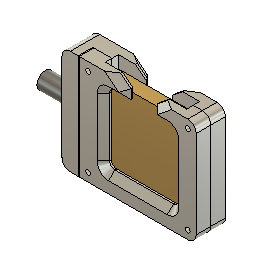
Elara 4th axis 0.5in jig (Autodesk Fusion 360 design; units mm, degrees)
Autodesk Fusion 360 part; units mm, degrees
note: some values were not read from the file. Set by a fixed rule: which sketch regions a step uses.
sketch "Sketch1" plane through (0, 0, 0) normal (0, 0, 1) x (1, 0, 0)
  line L0 (8, 0) -> (120.4, 0)
  line L1 (128.4, 8) -> (128.4, 92)
  line L2 (120.4, 100) -> (8, 100)
  line L3 (0, 92) -> (0, 8)
  circle A0 centre (72.7, 50) radius 23.3625 construction
  circle A1 centre (72.7, 50) radius 18.6 construction
  circle A2 centre (72.7, 50) radius 24
  line L4 (44.6, 83.1) -> (100.8, 83.1)
  line L5 (105.8, 78.1) -> (105.8, 21.9)
  line L6 (100.8, 16.9) -> (44.6, 16.9)
  line L7 (39.6, 21.9) -> (39.6, 78.1)
  arc A3 (128.4, 92) -> (120.4, 100) centre (120.4, 92) ccw
  arc A4 (120.4, 0) -> (128.4, 8) centre (120.4, 8) ccw
  circle A5 centre (120.4, 92) radius 1.65
  circle A6 centre (120.4, 8) radius 1.65
  circle A7 centre (25, 92) radius 1.65
  circle A8 centre (25, 8) radius 1.65
  line L8 (0, 50) -> (-50, 50) construction
  line L9 (60.2, 70.4878) -> (60.2, 100)
  line L10 (85.2, 70.4878) -> (85.2, 100)
  line L11 (72.7, 50) -> (72.7, 100) construction
  line L12 (16, 100) -> (16, 0)
  line L13 (0, 58) -> (-30, 58)
  line L14 (-30, 58) -> (-30, 50)
  line L15 (-30, 50) -> (0, 50)
  line L16 (33.8, 0) -> (33.8, 100)
  line L17 (111.6, 0) -> (111.6, 100)
  line L18 (15.5, 0) -> (15.5, 100)
  line L19 (16.5, 0) -> (16.5, 100)
  circle A9 centre (25, 92) radius 2.25
  circle A10 centre (120.4, 92) radius 2.25
  circle A11 centre (120.4, 8) radius 2.25
  circle A12 centre (25, 8) radius 2.25
  line L20 (60.2, 92) -> (50.2, 100)
  line L21 (85.2, 92) -> (95.2, 100)
  line L22 (34.6, 100) -> (34.6, 0)
  line L23 (110.8, 0) -> (110.8, 100)
  line L24 (33.8, 11.9) -> (111.6, 11.9)
  line L25 (33.8, 88.1) -> (111.6, 88.1)
  arc A13 (33.8, 11.9) -> (43.8, 11.9) centre (38.8, 11.9) ccw
  arc A14 (101.6, 11.9) -> (111.6, 11.9) centre (106.6, 11.9) ccw
  arc A15 (8, 100) -> (0, 92) centre (8, 92) ccw
  arc A16 (0, 8) -> (8, 0) centre (8, 8) ccw
  line L26 (103.9728, 65.6083) -> (118.9039, 65.6806) construction
  line L27 (118.9039, 65.6806) -> (118.8893, 68.6863) construction
  line L28 (118.8893, 68.6863) -> (103.9583, 68.614) construction
  line L29 (103.9583, 68.614) -> (103.9728, 65.6083) construction
  line L30 (0.7334, -6.4335) -> (20.3258, -6.3506) construction
  line L31 (20.3258, -6.3506) -> (20.3131, -3.3448) construction
  line L32 (20.3131, -3.3448) -> (0.7207, -3.4278) construction
  line L33 (0.7207, -3.4278) -> (0.7334, -6.4335) construction
  line L34 (-18.6738, 11.9015) -> (0.9186, 11.9844) construction
  line L35 (0.9186, 11.9844) -> (0.9059, 14.9901) construction
  line L36 (0.9059, 14.9901) -> (-18.6865, 14.9072) construction
  line L37 (-18.6865, 14.9072) -> (-18.6738, 11.9015) construction
  line L38 (-9.6516, 2.3848) -> (13.035, 2.4962) construction
  line L39 (13.035, 2.4962) -> (13.0067, 8.2636) construction
  line L40 (13.0067, 8.2636) -> (-9.6799, 8.1522) construction
  line L41 (-9.6799, 8.1522) -> (-9.6516, 2.3848) construction
  line L42 (0, 50) -> (22, 50) construction
  arc A17 (44.6, 83.1) -> (39.6, 78.1) centre (44.6, 78.1) ccw
  arc A18 (105.8, 78.1) -> (100.8, 83.1) centre (100.8, 78.1) ccw
  arc A19 (100.8, 16.9) -> (105.8, 21.9) centre (100.8, 21.9) ccw
  arc A20 (39.6, 21.9) -> (44.6, 16.9) centre (44.6, 21.9) ccw
  line L43 (0, 58) -> (14, 58)
  line L44 (14, 58) -> (14, 50)
  line L45 (0, 50) -> (14, 50)
  circle A21 centre (72.7, 50) radius 31.75 construction
  circle A22 centre (72.7, 50) radius 26.5 construction
  point P0 (0, 100)
  point P1 (39.6, 83.1)
  point P2 (105.8, 83.1)
  point P3 (105.8, 16.9)
  point P4 (39.6, 50)
  point P5 (72.7, 83.1)
  dimension "d1" = 37.2
  dimension "d3" = 4.7625
  dimension "d4" = 48
  dimension "d5" = 100
  dimension "d9" = 66.2
  dimension "d10" = 66.2
  dimension "d11" = 8
  dimension "d12" = 8
  dimension "d13" = 3.3
  dimension "d14" = 3.3
  dimension "d15" = 3.3
  dimension "d16" = 3.3
  dimension "d19" = 50
  dimension "d20" = 12.5
  dimension "d21" = 12.5
  dimension "d22" = 16.9
  dimension "d29" = 8
  dimension "d31" = 30
  dimension "d44" = 0.5
  dimension "d45" = 0.5
  dimension "d46" = 4.5
  dimension "d47" = 4.5
  dimension "d48" = 4.5
  dimension "d49" = 4.5
  dimension "d50" = 8
  dimension "d51" = 10
  dimension "d55" = 10
  dimension "d56" = 8
  dimension "d57" = 38.1
  dimension "d58" = 38.1
  dimension "d65" = 38.1
  dimension "d66" = 38.1
  dimension "d67" = 5
  dimension "d68" = 5
  dimension "d69" = 8
  dimension "d70" = 8
  dimension "d71" = 2
  dimension "d73" = 2
  dimension "d74" = 2
  dimension "d76" = 2
  dimension "d77" = 50
  dimension "d78" = 0.8
  dimension "d79" = 0.8
  dimension "d84" = 8.8
  dimension "d85" = 8.8
  dimension "d86" = 16
  dimension "d87" = 9
  dimension "d88" = 5
  dimension "d89" = 5
  dimension "d90" = 33.1
  dimension "d91" = 33.1
  dimension "d98" = 14
  dimension "d100" = 63.5
  dimension "d101" = 53
  constraint horizontal L0
  constraint vertical L1
  constraint horizontal L2
  constraint vertical L3
  constraint concentric A0 A1
  constraint concentric A1 A2
  constraint horizontal L4
  constraint vertical L5
  constraint horizontal L6
  constraint vertical L7
  constraint tangent L1 A3
  constraint tangent L2 A3
  constraint tangent L0 A4
  constraint tangent L1 A4
  constraint concentric A3 A5
  constraint concentric A4 A6
  constraint horizontal A3.centre A7.centre
  constraint horizontal A4.centre A8.centre
  constraint vertical A7.centre A8.centre
  constraint perpendicular L3 L8
  constraint vertical A0.centre P5
  constraint horizontal A0.centre P4
  constraint coincident A2 L9.start
  constraint coincident L2 L9.end
  constraint perpendicular L2 L9
  constraint coincident A2 L10.start
  constraint coincident L2 L10.end
  constraint perpendicular L2 L10
  constraint coincident A0.centre A1.centre
  constraint coincident L2 L11.end
  constraint perpendicular L2 L11
  constraint coincident L2 L12.start
  constraint coincident L0 L12.end
  constraint perpendicular L0 L12
  constraint coincident L3 L13.start
  constraint perpendicular L3 L13
  constraint coincident L8 L14.end
  constraint perpendicular L8 L14
  constraint coincident L0 L16.start
  constraint coincident L2 L16.end
  constraint perpendicular L2 L16
  constraint coincident L0 L17.start
  constraint coincident L2 L17.end
  constraint perpendicular L2 L17
  constraint coincident L0 L18.start
  constraint coincident L2 L18.end
  constraint perpendicular L2 L18
  constraint coincident L0 L19.start
  constraint coincident L2 L19.end
  constraint perpendicular L2 L19
  constraint concentric A7 A9
  constraint concentric A5 A10
  constraint concentric A6 A11
  constraint concentric A8 A12
  constraint coincident L9 L20.start
  constraint coincident L2 L20.end
  constraint coincident L10 L21.start
  constraint coincident L2 L21.end
  constraint coincident L2 L22.start
  constraint coincident L0 L22.end
  constraint perpendicular L0 L22
  constraint coincident L0 L23.start
  constraint coincident L2 L23.end
  constraint perpendicular L2 L23
  constraint coincident L16 L24.start
  constraint coincident L17 L24.end
  constraint perpendicular L17 L24
  constraint coincident L16 L25.start
  constraint coincident L17 L25.end
  constraint perpendicular L17 L25
  constraint tangent L16 A13
  constraint coincident L24 A13.end
  constraint tangent L17 A14
  constraint coincident L24 A14.start
  constraint coincident L3 L8.start
  constraint coincident P0 L2
  constraint coincident P0 L3
  constraint tangent L2 A15
  constraint tangent L3 A15
  constraint coincident origin L0
  constraint coincident origin L3
  constraint tangent L0 A16
  constraint tangent L3 A16
  constraint perpendicular L19 L42
  constraint coincident A0.centre L42
  constraint coincident L4 P5
  constraint coincident L7 P4
  constraint coincident P1 L4
  constraint coincident P1 L7
  constraint tangent L4 A17
  constraint tangent L7 A17
  constraint coincident P2 L4
  constraint coincident P2 L5
  constraint tangent L4 A18
  constraint tangent L5 A18
  constraint equal A17 A18
  constraint coincident P3 L5
  constraint coincident P3 L6
  constraint tangent L5 A19
  constraint tangent L6 A19
  constraint equal A17 A19
  constraint tangent L6 A20
  constraint tangent L7 A20
  constraint perpendicular L3 L43
  constraint coincident L42 L44.end
  constraint perpendicular L42 L44
  constraint concentric A2 A21
  measures "d1" diameter of A1
  measures "d3" distance of A0 A1
  measures "d4" diameter of A2
  measures "d5" distance of origin P0
  measures "d9" distance of P2 P3
  measures "d10" distance of P1 P2
  measures "d11" radius of A3
  measures "d12" radius of A4
  measures "d13" diameter of A6
  measures "d14" diameter of A5
  measures "d15" diameter of A7
  measures "d16" diameter of A8
  measures "d19" distance of L8.start L8.end
  measures "d20" distance of L9 L11
  measures "d21" distance of L10 L11
  measures "d22" distance of L2 L4
  measures "d29" distance of L8 L13
  measures "d31" distance of L13.start L13.end
  measures "d44" distance of L12 L19
  measures "d45" distance of L12 L18
  measures "d46" diameter of A12
  measures "d47" diameter of A11
  measures "d48" diameter of A10
  measures "d49" diameter of A9
  measures "d50" distance of L9.end L20.start
  measures "d51" distance of L9.end L20.end
  measures "d55" distance of L10.end L21.end
  measures "d56" distance of L10.end L21.start
  measures "d57" distance of L11 L22
  measures "d58" distance of L11 L23
  measures "d65" distance of A0.centre L24
  measures "d66" distance of A0.centre L25
  measures "d67" radius of A13
  measures "d68" radius of A14
  measures "d69" radius of A15
  measures "d70" radius of A16
  measures "d77" distance of origin L15
  measures "d78" distance of L16 L22
  measures "d79" distance of L17 L23
  measures "d84" distance of L17 A4.centre
  measures "d85" distance of A8.centre L16
  measures "d86" distance of L3 L12
  measures "d87" distance of L12 A8.centre
  measures "d88" radius of A17
  measures "d89" radius of A20
  measures "d90" distance of A0.centre L7
  measures "d91" distance of A0.centre L6
  measures "d98" distance of L3 L44
  measures "d100" diameter of A21
  measures "d101" diameter of A22
extrude "Extrude1" add sketch "Sketch1" against normal blind 14 contours L0 L2 L3 L18 A15 A16 L43 L44 L45 | L0 L2 L12 L18 | L0 L2 L12 L19 | L3 L43 L44 L45 | L0 L2 L16 L19 | L0 L16 L22 A13 | L0 L22 L23 L24 A13 A14 | L16 L22 L24 L25 | L22 L24 A13 | L2 L16 L22 L25 | L0 L17 L23 A14 | L22 L24 A13 | L4 L5 L6 L7 L9 L10 L22 L23 L24 L25 A17 A18 A19 A20 | L2 L9 L20 L22 L25 | L0 L1 L2 A3 A4 L17 | L23 L24 A14 | L23 L24 A14 | L17 L23 L24 L25 | L2 L17 L23 L25 | L2 L10 L21 L23 L25 | A9 | A10 | A11 | A12 makes body 1
extrude "Extrude2" add sketch "Sketch1" along normal blind 14 contours L0 L2 L3 L18 A15 A16 L43 L44 L45 | L3 L43 L44 L45 bodies 1
revolve "Revolve2" cut sketch "Sketch1" angle 360 about axis through (0, 50, 0) along (-1, 0, 0) contours L3 L43 L44 L45 bodies 1
revolve "Revolve1" add sketch "Sketch1" angle 360 about axis through (0, 50, 0) along (-1, 0, 0) separate body contours L3 L13 L14 L15 | L3 L43 L44 L45 makes body 2
fillet "Fillet1" [suppressed]
extrude "Extrude3" cut sketch "Sketch1" against normal blind 6.25 contours L16 L22 L24 L25 | L22 L24 A13 | L2 L16 L22 L25 | L22 L24 A13 | L4 L5 L6 L7 L9 L10 L22 L23 L24 L25 A17 A18 A19 A20 | L2 L9 L20 L22 L25 | L23 L24 A14 | L23 L24 A14 | L2 L9 L20 | L17 L23 L24 L25 | L2 L17 L23 L25 | L2 L10 L21 L23 L25 | A2 L4 L5 L6 L7 L9 L10 A17 A18 A19 A20 | L2 L10 L21 bodies 1
extrude "Extrude4" add sketch "Sketch1" along normal blind 14 separate body contours L0 L2 L16 L19 | L0 L16 L22 A13 | L0 L22 L23 L24 A13 A14 | L16 L22 L24 L25 | L22 L24 A13 | L2 L16 L22 L25 | L0 L17 L23 A14 | L22 L24 A13 | L4 L5 L6 L7 L9 L10 L22 L23 L24 L25 A17 A18 A19 A20 | L2 L9 L20 L22 L25 | L0 L1 L2 A3 A4 L17 | L23 L24 A14 | L23 L24 A14 | L17 L23 L24 L25 | L2 L17 L23 L25 | L2 L10 L21 L23 L25 makes body 3
extrude "Extrude5" cut sketch "Sketch1" along normal blind 6.25 contours L16 L22 L24 L25 | L22 L24 A13 | L2 L16 L22 L25 | L22 L24 A13 | L4 L5 L6 L7 L9 L10 L22 L23 L24 L25 A17 A18 A19 A20 | L2 L9 L20 L22 L25 | L23 L24 A14 | L23 L24 A14 | L2 L9 L20 | L17 L23 L24 L25 | L2 L17 L23 L25 | L2 L10 L21 L23 L25 | A2 L4 L5 L6 L7 L9 L10 A17 A18 A19 A20 | L2 L10 L21 bodies 3
chamfer "Chamfer1" distance 6 angle 45 26 edges at (90.2, 96, -14) (85.2, 87.55, -14) (93, 83.1, -14) (52.4, 83.1, -14) (41.0645, 81.6355, -14) (39.6, 50, -14) (41.0645, 18.3645, -14) (72.7, 16.9, -14) (104.3355, 18.3645, -14) (105.8, 50, -14) (104.3355, 81.6355, -14) (60.2, 87.55, -14) (55.2, 96, -14) (55.2, 96, 14) (60.2, 87.55, 14) (52.4, 83.1, 14) (93, 83.1, 14) (104.3355, 81.6355, 14) (105.8, 50, 14) (104.3355, 18.3645, 14) (72.7, 16.9, 14) (41.0645, 18.3645, 14) (39.6, 50, 14) (41.0645, 81.6355, 14) (85.2, 87.55, 14) (90.2, 96, 14) on bodies 1 3
extrude "Extrude6" add sketch "Sketch1" along normal blind 6.35 and the other way blind 6.35 separate body contours L4 L5 L6 L7 L9 L10 L22 L23 L24 L25 A17 A18 A19 A20 | L4 L9 L10 L25 | A2 L4 L5 L6 L7 L9 L10 A17 A18 A19 A20 | A2 L4 L9 L10 | A2 makes body 4
equation "d3 = 0.125 in + 0.0625 in"
